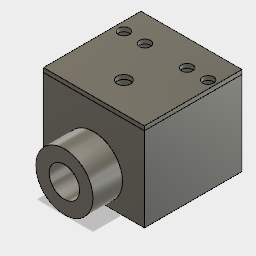
04_audiojack v4 (Autodesk Fusion 360 design; units mm, degrees)
Autodesk Fusion 360 part; units mm, degrees
sketch "Sketch1" plane through (0, 0, 0) normal (0, 1, 0) x (1, 0, 0)
  line L0 (-6.067, 6.1) -> (5.933, 6.1)
  line L1 (5.933, 6.1) -> (5.933, -5.5)
  line L2 (5.933, -5.5) -> (-6.067, -5.5)
  line L3 (-6.067, -5.5) -> (-6.067, 6.1)
  line L4 (-3.467, -5.5) -> (3.433, -5.5)
  line L5 (3.433, -5.5) -> (3.433, -9)
  line L6 (3.433, -9) -> (-3.467, -9)
  line L7 (-3.467, -9) -> (-3.467, -5.5)
  circle A0 centre (5, 3) radius 0.65
  circle A1 centre (5, 3) radius 0.65
  circle A2 centre (2.5, 3) radius 0.65
  circle A3 centre (-2.5, 3) radius 0.65
  circle A4 centre (-5, 3) radius 0.65
  circle A5 centre (0, -2) radius 0.8
  point P0 (5, 3)
  point P1 (0, 3)
  dimension "d1" = 11.6
  dimension "d2" = 12
  dimension "d3" = 3.5
  dimension "d4" = 6.9
  dimension "d5" = 2.6
  dimension "d9" = 1.3
  dimension "d10" = 8.5
  dimension "d14" = 5
  dimension "d15" = 1.3
  dimension "d16" = 1.3
  dimension "d17" = 1.3
  dimension "d18" = 1.3
  dimension "d19" = 1.6
  dimension "d20" = 5
  dimension "d21" = 7
  measures "d1" distance of L0.start L2.end
  measures "d2" distance of L0.start L0.end
  measures "d3" distance of L4.start L6.end
  measures "d4" distance of L5.end L6.end
  measures "d5" distance of L2.end L7
  measures "d9" diameter of A0
  measures "d10" distance of L2 P0
  measures "d14" distance of P0 P1
  measures "d15" diameter of A1
  measures "d16" diameter of A2
  measures "d17" diameter of A3
  measures "d18" diameter of A4
  measures "d19" diameter of A5
  measures "d20" distance of P1 A5.centre
  measures "d21" distance of L6 A5.centre
extrude "Extrude1" add sketch "Sketch1" along normal blind 10 contours L0 L1 L2 L3 L4 makes body 1
sketch "Sketch2" plane through (0, 0, 5.5) normal (0, 0, 1) x (1, 0, 0)
  line L0 (-6.067, 0) -> (5.933, 0)
  line L1 (5.933, 0) -> (5.933, 10)
  line L2 (5.933, 10) -> (-6.067, 10)
  line L3 (-6.067, 10) -> (-6.067, 0)
  circle A0 centre (-0.067, 3.5) radius 3.4
  circle A1 centre (-0.067, 3.5) radius 1.8
  dimension "d24" = 6.8
  dimension "d25" = 6
  dimension "d26" = 6.5
  dimension "d27" = 3.6
  measures "d24" diameter of A0
  measures "d25" distance of L3 A0.centre
  measures "d26" distance of L2 A0.centre
  measures "d27" diameter of A1
extrude "Extrude2" add sketch "Sketch2" along normal blind 3.5 contours A0 bodies 1
extrude "Extrude3" cut 1 faces at (-0.4869, 3.3582, 5.5) along direction (0, 0, -1) blind 5 on bodies 1 bodies 1
extrude "Extrude4" add 1 faces at (-3.9395, 10, 1.7161) along direction (0, 1, 0) blind 0.5 separate body on bodies 1 makes body 2
